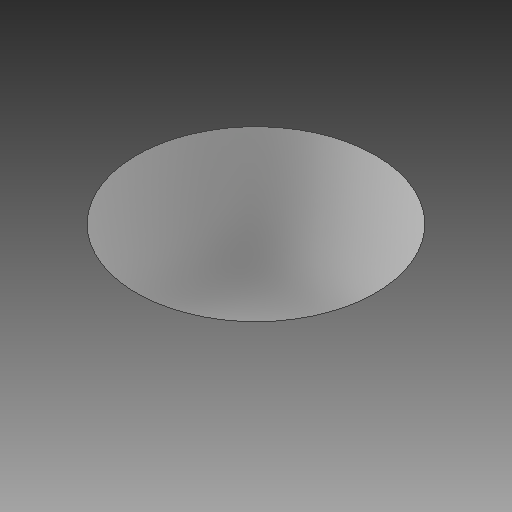
# Autodesk Inventor part: mirror
Saved by Autodesk Inventor 2020 (Build 240168000, 168)
## iProperties
Created: 2024-11-25
Part Number: mirror
Material: Стекло
Document SubType Name: Modeling
Designer: Ivan
Density: 2.18 g/cm^3
Appearance: Хром — полированный
Mass: 84.4212 g
Surface Area: 122.151 cm^2
Volume: 38.7253 cm^3
Author: Ivan
Autodesk Inventor part; units mm, degrees
ref_plane "YZ Plane" through (0, 0, 0) normal (1, 0, 0) x (0, 1, 0)
ref_plane "XZ Plane" through (0, 0, 0) normal (0, 1, 0) x (-1, 0, 0)
ref_plane "XY Plane" through (0, 0, 0) normal (0, 0, 1) x (1, 0, 0)
sketch "Эскиз1" plane through (0, 0, 0) normal (1, 0, 0) x (0, 1, 0)
  line L0 (0, 0) -> (0, -43)
  line L1 (0, -43) -> (-20, 0)
  line L2 (-20, 0) -> (0, 0)
  arc A0 (-19.85, 0) -> (-19.7028, -0.6391) centre (-18.2691, 0.0277) ccw
  dimension "d0" = 20
  dimension "d1" = 43
  dimension "d3" = 0.15
  constraints: 6 end point, 2 point on circle, 2 point on line, 1 centre point, 1 horizontal, 1 perpendicular, 1 tangent
  measures "d0" distance of L1.end L0.start
  measures "d1" distance of L0.start L0.end
  measures "d3" distance of A0.start L1.end
revolve "Вращение1" add sketch "Эскиз1" angle 360 about axis through (0, -20, 0) along (0, 1, 0) contours L0 L1 A0 L2
